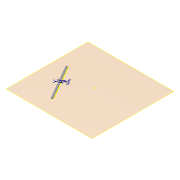
# Autodesk Inventor part: led
Saved by Autodesk Inventor 2014 (Build 180170000, 170)
## iProperties
Created: 2016-05-23
Part Number: led
Material: Generic
Document SubType Name: Modeling
Designer: admin
Density: 1 g/cm^3
Appearance: Default
Author: admin
Autodesk Inventor part; units mm, degrees
ref_plane "YZ Plane" through (0, 0, 0) normal (1, 0, 0) x (0, 1, 0)
ref_plane "XZ Plane" through (0, 0, 0) normal (0, 1, 0) x (-1, 0, 0)
ref_plane "XY Plane" through (0, 0, 0) normal (0, 0, 1) x (1, 0, 0)
ref_plane "Work Plane1" through (0, 0, 0) normal (0, 0, 1) x (1, 0, 0)
sketch "Sketch1" plane through (0, 0, 0) normal (0, 0, 1) x (1, 0, 0)
  line L0 (-103.308954, -65.418955) -> (-101.576903, -64.418955)
  line L1 (-106.576903, -55.758701) -> (-108.308954, -56.758701)
  line L2 (-107.442928, -56.258701) -> (-102.442928, -64.918955)
  line L3 (-159.3979, 23.432932) -> (-59.140775, -149.623444)
  line L4 (-59.140775, -149.623444) -> (-50.487957, -144.610587)
  line L5 (-50.487957, -144.610587) -> (-150.745081, 28.445788)
  line L6 (-150.745081, 28.445788) -> (-159.3979, 23.432932)
  line L7 (-159.3979, 23.432932) -> (-50.487957, -144.610587) construction
  line L8 (-59.140775, -149.623444) -> (-150.745081, 28.445788) construction
  point P0 (0, 0)
  point P1 (-104.942928, -60.588828)
  dimension "d12" = 10
  dimension "d13" = 200
  constraints: 14 end point, 5 midpoint, 2 parallel, 1 perpendicular
  measures "d12" distance between parallel lines of L3 L5
  measures "d13" distance between parallel lines of L4 L6
sketch "Sketch1 outline for Extrusion1" plane through (0, 0, 0) normal (0, 0, 1) x (1, 0, 0)
  line L0 (-150.745081, 28.445788) -> (-159.3979, 23.432932)
  line L1 (-50.487957, -144.610587) -> (-150.745081, 28.445788)
  line L2 (-59.140775, -149.623444) -> (-50.487957, -144.610587)
  line L3 (-159.3979, 23.432932) -> (-59.140775, -149.623444)
extrude "Extrusion1" add sketch "Sketch1 outline for Extrusion1" along normal blind 1
sketch "Sketch2" plane through (0, 0, 0) normal (0, 0, -1) x (-1, 0, 0)
  line L0 (159.3979, 23.432932) -> (59.140775, -149.623444)
  line L1 (50.487957, -144.610587) -> (150.745081, 28.445788)
  line L2 (105.274591, -54.031725) -> (107.781019, -49.705316)
  line L3 (107.781019, -49.705316) -> (112.97271, -52.713029)
  line L4 (112.97271, -52.713029) -> (110.466282, -57.039439)
  line L5 (110.466282, -57.039439) -> (105.274591, -54.031725)
  line L6 (105.274591, -54.031725) -> (112.97271, -52.713029) construction
  line L7 (107.781019, -49.705316) -> (110.466282, -57.039439) construction
  line L8 (109.269338, -63.095256) -> (100.616519, -58.0824)
  line L9 (109.269338, -63.095256) -> (100.616519, -58.0824)
  line L10 (134.333619, -19.831162) -> (125.6808, -14.818306)
  line L11 (121.324129, -38.297433) -> (118.8177, -42.623843)
  line L12 (118.8177, -42.623843) -> (113.626009, -39.616129)
  line L13 (113.626009, -39.616129) -> (116.132437, -35.289719)
  line L14 (116.132437, -35.289719) -> (121.324129, -38.297433)
  line L15 (129.675547, -23.881837) -> (127.169119, -28.208247)
  line L16 (127.169119, -28.208247) -> (121.977428, -25.200533)
  line L17 (121.977428, -25.200533) -> (124.483856, -20.874123)
  line L18 (124.483856, -20.874123) -> (129.675547, -23.881837)
  line L19 (120.070915, -40.460638) -> (114.879223, -37.452924)
  line L20 (128.422333, -26.045042) -> (123.230642, -23.037328)
  point P0 (0, 0)
  point P1 (109.12365, -53.372377)
  dimension "d3" = 5
  dimension "d10" = 2
  dimension "d11" = 2
  dimension "d14" = 50
  dimension "d15" = 2
  dimension "d16" = 2
  dimension "d17" = 2
  dimension "d18" = 2
  dimension "d19" = 5
  dimension "d20" = 5
  dimension "d23" = 25
  dimension "d26" = 16.66
  dimension "d27" = 16.66
  constraints: 38 end point, 9 parallel, 8 midpoint, 5 perpendicular, 2 point on line
  measures "d3" distance between parallel lines of L5 L3
  measures "d10" distance between parallel lines of L0 L4
  measures "d11" distance between parallel lines of L1 L2
  measures "d14" distance between parallel lines of L9 L10
  measures "d15" distance between parallel lines of L1 L17
  measures "d16" distance between parallel lines of L0 L15
  measures "d17" distance between parallel lines of L0 L11
  measures "d18" distance between parallel lines of L1 L13
  measures "d19" distance between parallel lines of L12 L14
  measures "d20" distance between parallel lines of L16 L18
  measures "d23" distance between parallel lines of L10 L19
  measures "d26" distance from line of point (109.124, -53.372) L19
  measures "d27" distance between parallel lines of L19 L20
sketch "Sketch2 outline for Extrusion2" plane through (0, 0, 0) normal (0, 0, -1) x (-1, 0, 0)
  line L0 (121.324129, -38.297433) -> (116.132437, -35.289719)
  line L1 (116.132437, -35.289719) -> (113.626009, -39.616129)
  line L2 (113.626009, -39.616129) -> (118.8177, -42.623843)
  line L3 (118.8177, -42.623843) -> (121.324129, -38.297433)
  line L4 (129.675547, -23.881837) -> (124.483856, -20.874123)
  line L5 (124.483856, -20.874123) -> (121.977428, -25.200533)
  line L6 (121.977428, -25.200533) -> (127.169119, -28.208247)
  line L7 (127.169119, -28.208247) -> (129.675547, -23.881837)
  line L8 (105.274591, -54.031725) -> (107.781019, -49.705316)
  line L9 (107.781019, -49.705316) -> (112.97271, -52.713029)
  line L10 (112.97271, -52.713029) -> (110.466282, -57.039439)
  line L11 (110.466282, -57.039439) -> (105.274591, -54.031725)
extrude "Extrusion2" add sketch "Sketch2 outline for Extrusion2" along normal blind 2 separate body
pattern_linear "Rectangular Pattern1" count 4 spacing 50 along (0.5012856, -0.8652819, 0) of "Extrusion2" first direction both ways yes bodies 2
sketch "Sketch3" plane through (0, 0, 1) normal (0, 0, 1) x (1, 0, 0)
  line L0 (-159.3979, 23.432932) -> (-59.140775, -149.623444)
  line L1 (-59.140775, -149.623444) -> (-50.487957, -144.610587)
  line L2 (-50.487957, -144.610587) -> (-150.745081, 28.445788)
  line L3 (-57.842853, -148.871515) -> (-52.842853, -157.531769) construction
  line L4 (-58.275865, -149.121515) -> (-53.275865, -157.781769)
  line L5 (-52.40984, -157.281769) -> (-57.40984, -148.621515)
  arc A0 (-57.40984, -148.621515) -> (-58.275865, -149.121515) centre (-57.842853, -148.871515) ccw
  arc A1 (-53.275865, -157.781769) -> (-52.40984, -157.281769) centre (-52.842853, -157.531769) ccw
  line L6 (-57.842853, -148.871515) -> (-47.842853, -148.871515) construction
  line L7 (-55.679648, -147.618301) -> (-50.666792, -156.27112) construction
  line L8 (-56.112289, -147.868944) -> (-51.099433, -156.521763)
  line L9 (-50.234151, -156.020477) -> (-55.247007, -147.367658)
  arc A2 (-55.247007, -147.367658) -> (-56.112289, -147.868944) centre (-55.679648, -147.618301) ccw
  arc A3 (-51.099433, -156.521763) -> (-50.234151, -156.020477) centre (-50.666792, -156.27112) ccw
  line L10 (-53.949084, -146.61573) -> (-48.949084, -155.275984) construction
  line L11 (-54.382097, -146.86573) -> (-49.382097, -155.525984)
  line L12 (-48.516072, -155.025984) -> (-53.516072, -146.36573)
  arc A4 (-53.516072, -146.36573) -> (-54.382097, -146.86573) centre (-53.949084, -146.61573) ccw
  arc A5 (-49.382097, -155.525984) -> (-48.516072, -155.025984) centre (-48.949084, -155.275984) ccw
  line L13 (-53.949084, -146.61573) -> (-43.949084, -146.61573) construction
  line L14 (-51.78588, -145.362516) -> (-46.78588, -154.02277) construction
  line L15 (-52.218892, -145.612516) -> (-47.218892, -154.27277)
  line L16 (-46.352867, -153.77277) -> (-51.352867, -145.112516)
  arc A6 (-51.352867, -145.112516) -> (-52.218892, -145.612516) centre (-51.78588, -145.362516) ccw
  arc A7 (-47.218892, -154.27277) -> (-46.352867, -153.77277) centre (-46.78588, -154.02277) ccw
  line L17 (-51.78588, -145.362516) -> (-41.78588, -145.362516) construction
  point P0 (0, 0)
  point P1 (-55.342853, -153.201642)
  point P2 (-53.17322, -151.944711)
  point P3 (-51.449084, -150.945857)
  point P4 (-49.28588, -149.692643)
  dimension "d33" = 60
  dimension "d34" = 1
  dimension "d35" = 10
  dimension "d36" = 1
  dimension "d37" = 60
  dimension "d38" = 1
  dimension "d39" = 60
  dimension "d40" = 1
  dimension "d41" = 1.5
  dimension "d42" = 1.5
  dimension "d43" = 10
  dimension "d44" = 4
  dimension "d45" = 4
  dimension "d46" = 10
  dimension "d47" = 10
  constraints: 38 end point, 16 point on circle, 16 tangent, 8 centre point, 4 midpoint, 4 parallel, 4 point on line, 3 equal length, 3 horizontal, 1 perpendicular
  measures "d33" angle of L3 L6
  measures "d34" diameter of A1
  measures "d35" distance of L3.end L3.start
  measures "d36" diameter of A3
  measures "d37" angle of L10 L13
  measures "d38" diameter of A5
  measures "d39" angle of L14 L17
  measures "d40" diameter of A7
  measures "d41" distance from line of L0 L3.start
  measures "d42" distance from line of L2 L14.start
  measures "d43" distance of L7.end L7.start
  measures "d44" distance from line of L0 L7.start
  measures "d45" distance from line of L2 L10.start
  measures "d46" distance of L10.start L10.end
  measures "d47" distance of L14.end L14.start
sketch "Sketch3 outline for Extrusion3" plane through (0, 0, 1) normal (0, 0, 1) x (1, 0, 0)
  arc A0 (-57.40984, -148.621515) -> (-58.275865, -149.121515) centre (-57.842853, -148.871515) ccw
  line L0 (-52.40984, -157.281769) -> (-57.40984, -148.621515)
  arc A1 (-53.275865, -157.781769) -> (-52.40984, -157.281769) centre (-52.842853, -157.531769) ccw
  line L1 (-58.275865, -149.121515) -> (-53.275865, -157.781769)
  arc A2 (-55.247007, -147.367658) -> (-56.112289, -147.868944) centre (-55.679648, -147.618301) ccw
  line L2 (-50.234151, -156.020477) -> (-55.247007, -147.367658)
  arc A3 (-51.099433, -156.521763) -> (-50.234151, -156.020477) centre (-50.666792, -156.27112) ccw
  line L3 (-56.112289, -147.868944) -> (-51.099433, -156.521763)
  arc A4 (-53.516072, -146.36573) -> (-54.382097, -146.86573) centre (-53.949084, -146.61573) ccw
  line L4 (-48.516072, -155.025984) -> (-53.516072, -146.36573)
  arc A5 (-49.382097, -155.525984) -> (-48.516072, -155.025984) centre (-48.949084, -155.275984) ccw
  line L5 (-54.382097, -146.86573) -> (-49.382097, -155.525984)
  arc A6 (-51.352867, -145.112516) -> (-52.218892, -145.612516) centre (-51.78588, -145.362516) ccw
  line L6 (-46.352867, -153.77277) -> (-51.352867, -145.112516)
  arc A7 (-47.218892, -154.27277) -> (-46.352867, -153.77277) centre (-46.78588, -154.02277) ccw
  line L7 (-52.218892, -145.612516) -> (-47.218892, -154.27277)
extrude "Extrusion3" add sketch "Sketch3 outline for Extrusion3" along normal blind 1 separate body
fillet "Fillet1" radius 0.5 16 edges at (-46.5359, -154.4558, 2) (-48.8529, -149.4426, 2) (-52.0359, -144.9295, 2) (-49.7189, -149.9426, 2) (-48.6991, -155.709, 2) (-51.0161, -150.6959, 2) (-54.1991, -146.1827, 2) (-51.8821, -151.1959, 2) (-50.4161, -156.7038, 2) (-52.7406, -151.6941, 2) (-55.9303, -147.1857, 2) (-53.6059, -152.1954, 2) (-52.5929, -157.9648, 2) (-54.9098, -152.9516, 2) (-58.0929, -148.4385, 2) (-55.7759, -153.4516, 2)
body "Solid1"
body "Solid2"
body "Solid3"
